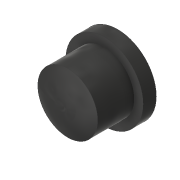
# Autodesk Inventor part: Button Piece Large
Saved by Autodesk Inventor 2017 (Build 210142000, 142)
## iProperties
Created: 2016-08-11
Part Number: Button Piece Large
Material: Generic
Document SubType Name: Modeling
Designer: ge937963
Density: 1 g/cm^3
Appearance: Fine Textured - Black
Mass: 0.169063 g
Surface Area: 1.89017 cm^2
Volume: 0.169063 cm^3
Author: ge937963
Autodesk Inventor part; units mm, degrees
ref_plane "YZ Plane" through (0, 0, 0) normal (1, 0, 0) x (0, 1, 0)
ref_plane "XZ Plane" through (0, 0, 0) normal (0, 1, 0) x (-1, 0, 0)
ref_plane "XY Plane" through (0, 0, 0) normal (0, 0, 1) x (1, 0, 0)
sketch "Sketch1" plane through (0, 0, 0) normal (1, 0, 0) x (0, 1, 0)
  line L0 (-3.175, 3.9727) -> (-3.175, 2.3852)
  line L1 (3.175, 3.9727) -> (3.175, 2.3852)
  line L2 (8.5884, 3.9727) -> (-47.5777, 3.9727) projected
  line L3 (-47.5777, 2.3852) -> (8.5884, 2.3852) projected
  line L4 (-1.7526, -0.508) -> (-1.7526, 0)
  line L5 (1.7526, -0.508) -> (1.7526, 0)
  line L6 (1.7526, 0) -> (-1.7526, 0) projected
  line L7 (0, -1.3409) -> (0, 5.0091)
  line L8 (0, -1.3409) -> (-4.4284, -1.3409)
  line L9 (-4.4284, -1.3409) -> (-4.4284, 0.1831)
  line L10 (-4.4284, 0.1831) -> (-3.429, 0.1831)
  line L11 (-3.429, 0.1831) -> (-3.429, 4.3908)
  arc A0 (0, 5.0091) -> (-3.429, 4.3908) centre (0, -4.8085) ccw
  line L12 (0, 5.0091) -> (-0.228, 5.0091)
  point P0 (0, 0)
  point P1 (0, 0)
  dimension "d0" = 3.429
  dimension "d2" = 6.35
  dimension "d3" = 1.524
  constraints: 20 end point, 5 vertical, 3 perpendicular, 2 horizontal, 2 point on circle, 1 centre point, 1 midpoint, 1 tangent, 1 vertical alignment, 8 other
  measures "d0" distance between parallel lines of L11 L7
  measures "d2" distance of L7.start L7.end
  measures "d3" distance of L8.end L9.end
revolve "Revolution1" add sketch "Sketch1" angle 360 about axis through (0, 0, -1.3409) along (0, 0, 1) contours L2 L7 L3 L0 | L2 L11 A0 L7 | L0 L3 L11 L2 | L3 L7 L8 L9 L10 L11
body "Solid1"
